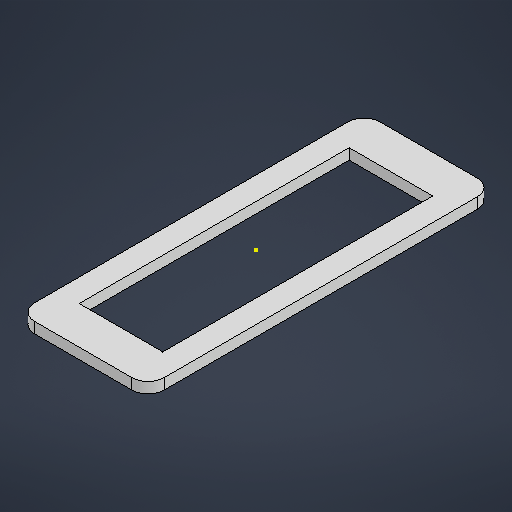
# Autodesk Inventor part: bottom
Saved by Autodesk Inventor 2026 (Build 300175050, 175E)
## iProperties
Created: 2025-09-05
Part Number: bottom
Material: 一般
Document SubType Name: Modeling
Designer: ka0n7
Density: 1 g/cm^3
Appearance: 既定
Author: ka0n7
Autodesk Inventor part; units mm, degrees
ref_plane "YZ Plane" through (0, 0, 0) normal (1, 0, 0) x (0, 1, 0)
ref_plane "XZ Plane" through (0, 0, 0) normal (0, 1, 0) x (-1, 0, 0)
ref_plane "XY Plane" through (0, 0, 0) normal (0, 0, 1) x (1, 0, 0)
sketch "スケッチ1" plane through (0, 0, 0) normal (0, 1, 0) x (-1, 0, 0)
  line L0 (12, 32) -> (-12, 32)
  line L1 (-12, 32) -> (-12, -32)
  line L2 (-12, -32) -> (12, -32)
  line L3 (12, -32) -> (12, 32)
  line L4 (12, 32) -> (-12, -32) construction
  line L5 (-12, 32) -> (12, -32) construction
  line L6 (7.75, 25) -> (-7.75, 25)
  line L7 (-7.75, 25) -> (-7.75, -25)
  line L8 (-7.75, -25) -> (7.75, -25)
  line L9 (7.75, -25) -> (7.75, 25)
  line L10 (7.75, 25) -> (-7.75, -25) construction
  line L11 (-7.75, 25) -> (7.75, -25) construction
  point P0 (0, 0)
  dimension "d0" = 24
  dimension "d1" = 64
  dimension "d2" = 15.5
  dimension "d3" = 50
  constraints: 24 end point, 4 midpoint, 4 parallel, 2 horizontal, 2 perpendicular
  measures "d0" distance of L2.end L1.end
  measures "d1" distance of L2.end L0.start
  measures "d2" distance of L7.end L8.end
  measures "d3" distance of L8.end L6.start
extrude "押し出し1" add sketch "スケッチ1" along normal blind 2
sketch "スケッチ2" plane through (0, 2, 0) normal (0, 1, 0) x (1, 0, 0)
  point P0 (0, 0)
fillet "フィレット1" radius 3 4 edges at (-12, 1, 32) (12, 1, 32) (12, 1, -32) (-12, 1, -32)
